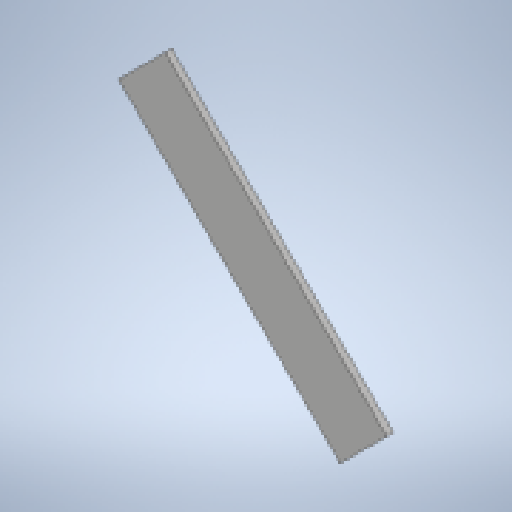
# Autodesk Inventor part: CameraPlate
Saved by Autodesk Inventor 2025.1 (Build 291241000, 241)
## iProperties
Created: 2025-06-16
Part Number: CameraPlate
Material: Generic
Document SubType Name: Modeling
Designer: User
Density: 1 g/cm^3
Appearance: Default
Author: User
Autodesk Inventor part; units mm, degrees
ref_plane "YZ Plane" through (0, 0, 0) normal (1, 0, 0) x (0, 1, 0)
ref_plane "XZ Plane" through (0, 0, 0) normal (0, 1, 0) x (-1, 0, 0)
ref_plane "XY Plane" through (0, 0, 0) normal (0, 0, 1) x (1, 0, 0)
sketch "Sketch3" plane through (0, 0, 0) normal (0, 0, 1) x (1, 0, 0)
  line L0 (-94.6243, 4.4908) -> (-47.5665, 51.5485) projected
  line L1 (-48.2912, 50.8239) -> (-38.3917, 60.7234) projected
  line L2 (-39.1164, 59.9987) -> (15.6159, 114.7309) projected
  line L3 (75.9757, -27.3497) -> (-17.6132, -120.9386) projected
  line L4 (-13.085, -29.4897) -> (-26.753, -15.8218) projected
  line L5 (-9.5495, -25.9542) -> (-23.2174, -12.2862)
  line L6 (33.9109, -69.4145) -> (-67.3094, 31.8057)
  line L7 (-67.3094, 31.8057) -> (-46.0962, 53.0189)
  line L8 (-46.0962, 53.0189) -> (55.1241, -48.2013)
  line L9 (55.1241, -48.2013) -> (33.9109, -69.4145)
  point P0 (0, 0)
  point P1 (55.1241, -48.2013)
  dimension "d0" = 5
  dimension "d1" = 30
  constraints: 10 end point, 3 parallel, 2 perpendicular, 2 point on line
  measures "d0" distance between parallel lines of L4 L5
  measures "d1" distance of L6.end L7.end
extrude "Extrusion1" add sketch "Sketch3" along normal blind 3
sketch "Sketch4" plane through (0, 0, 3) normal (0, 0, 1) x (1, 0, 0)
  line L0 (-37.1973, -4.3252) -> (-44.2684, 2.7459) projected
  line L1 (4.8755, -46.3981) -> (-2.1956, -39.327) projected
  line L2 (-67.3094, 31.8057) -> (33.9109, -69.4145) projected
  line L3 (-13.085, -29.4897) -> (-26.753, -15.8218) projected
  line L4 (-44.125, 2.6025) -> (-37.1973, -4.3252)
  line L5 (-37.1973, -4.3252) -> (-34.1879, -1.3158)
  line L6 (-34.1879, -1.3158) -> (-41.1156, 5.6119)
  line L7 (-41.1156, 5.6119) -> (-44.125, 2.6025)
  line L8 (-2.1956, -39.327) -> (4.8755, -46.3981)
  line L9 (4.8755, -46.3981) -> (7.8849, -43.3886)
  line L10 (7.8849, -43.3886) -> (0.8139, -36.3176)
  line L11 (0.8139, -36.3176) -> (-2.1956, -39.327)
  point P0 (0, 0)
  constraints: 16 end point, 4 parallel, 2 collinear, 2 perpendicular, 1 point on line
extrude "Extrusion2" add sketch "Sketch4" against normal up to surface (3 mm away)
sketch "Sketch5" plane through (0, 0, 3) normal (0, 0, 1) x (1, 0, 0)
  line L0 (-19.5198, 27.4945) -> (-12.4488, 20.4234) projected
  line L1 (22.553, -14.5784) -> (29.6241, -21.6495) projected
  line L2 (55.1241, -48.2013) -> (-46.0962, 53.0189) projected
  line L3 (-12.4488, 20.4234) -> (-19.5198, 27.4945)
  line L4 (-19.5198, 27.4945) -> (-20.0458, 26.9685)
  line L5 (-20.0458, 26.9685) -> (-12.9747, 19.8974)
  line L6 (-12.9747, 19.8974) -> (-12.4488, 20.4234)
  line L7 (29.6241, -21.6495) -> (22.553, -14.5784)
  line L8 (22.553, -14.5784) -> (22.0271, -15.1043)
  line L9 (22.0271, -15.1043) -> (29.0981, -22.1754)
  line L10 (29.0981, -22.1754) -> (29.6241, -21.6495)
  point P0 (0, 0)
  constraints: 16 end point, 5 parallel, 2 perpendicular, 1 collinear
extrude "Extrusion3" add sketch "Sketch5" against normal up to surface (3 mm away)
sketch "Sketch6" plane through (0, 0, 3) normal (0, 0, 1) x (1, 0, 0)
  ellipse E0 centre (-19.5198, 20.4234) end of major axis (-20.5805, 21.4841) minor radius 1.5 projected
  ellipse E1 centre (-37.1974, 2.7458) end of major axis (-38.258, 3.8065) minor radius 1.5 projected
  ellipse E2 centre (22.5531, -21.6494) end of major axis (21.4924, -20.5888) minor radius 1.5 projected
  ellipse E3 centre (4.8755, -39.327) end of major axis (3.8148, -38.2663) minor radius 1.5 projected
  point P0 (0, 0)
  constraints: 4 other
extrude "Extrusion4" cut sketch "Sketch6" against normal blind 10
sketch "Sketch8" plane through (0, 0, 0) normal (0, 0, -1) x (-1, 0, 0)
  line L0 (53.1672, 45.9478) -> (-48.053, -55.2724)
  line L1 (60.2383, 38.8768) -> (-40.9819, -62.3435)
  line L2 (61.0868, 38.0282) -> (-40.1334, -63.192)
  line L3 (59.3898, 39.7253) -> (-41.8305, -61.4949)
  line L4 (52.3187, 46.7964) -> (-48.9015, -54.4239)
  line L5 (54.0158, 45.0993) -> (-47.2045, -56.1209)
  line L6 (61.0868, 38.0282) -> (59.3898, 39.7253)
  line L7 (54.0158, 45.0993) -> (52.3187, 46.7964)
  line L8 (-40.1334, -63.192) -> (-41.8305, -61.4949)
  line L9 (-47.2045, -56.1209) -> (-48.9015, -54.4239)
  line L10 (-33.9109, -69.4145) -> (-55.1241, -48.2013) projected
  point P0 (0, 0)
  point P1 (46.0962, 53.0189)
  point P2 (67.3094, 31.8057)
  dimension "d16" = 1.2
  dimension "d17" = 1.2
  dimension "d18" = 1.2
  dimension "d19" = 1.2
  constraints: 20 end point, 4 parallel, 2 collinear, 2 perpendicular
  measures "d16" distance between parallel lines of L1 L2
  measures "d17" distance between parallel lines of L1 L3
  measures "d18" distance between parallel lines of L0 L4
  measures "d19" distance between parallel lines of L0 L5
extrude "Extrusion6" add sketch "Sketch8" along normal blind 5
chamfer "Chamfer1" distance 0.73 angle 45 4 edges at (29.0981, -22.1754, 1.5) (22.0271, -15.1043, 1.5) (-20.0458, 26.9685, 1.5) (-12.9747, 19.8974, 1.5)
chamfer "Chamfer2" distance 4.25 angle 45 4 edges at (-41.1156, 5.6119, 1.5) (-34.1879, -1.3158, 1.5) (7.8849, -43.3886, 1.5) (0.8139, -36.3176, 1.5)
sketch "Sketch9" plane through (-67.3094, 31.8057, 0) normal (-0.7071068, 0.7071068, 0) x (-0.7071068, -0.7071068, 0)
  line L0 (-30, 0) -> (-21.2, 0) projected
  line L1 (-21.2, 0) -> (-21.2, -5) projected
  line L2 (-18.8, -5) -> (-21.2, -5) projected
  line L3 (-18.8, 0) -> (-18.8, -5) projected
  line L4 (-18.8, 0) -> (-11.2, 0) projected
  line L5 (-11.2, 0) -> (-11.2, -5) projected
  line L6 (-8.8, -5) -> (-11.2, -5) projected
  line L7 (-8.8, 0) -> (-8.8, -5) projected
  line L8 (-8.8, 0) -> (0, 0) projected
  line L9 (0, 0) -> (0, 3) projected
  line L10 (-30, 3) -> (0, 3) projected
  line L11 (-30, 0) -> (-30, 3) projected
  line L12 (-30, 3) -> (0, 3)
  line L13 (0, 3) -> (0, 0)
  line L14 (0, 0) -> (-30, 0)
  line L15 (-30, 0) -> (-30, 3)
  point P0 (-25.1049, 0)
  constraints: 8 end point, 2 parallel, 1 horizontal, 1 perpendicular
extrude "Extrusion7" add sketch "Sketch9" along normal blind 13 contours L11 L10 L9 L8 L14 L4 L0
sketch "Sketch10" plane through (55.1241, -48.2013, 3) normal (0.7071068, -0.7071068, 0) x (-0.7071068, -0.7071068, 0)
  line L0 (30, 3) -> (30, 0) projected
  line L1 (0, 3) -> (-0.73, 3) projected
  line L2 (30, 0) -> (-0.73, 0)
  line L3 (-0.73, 0) -> (-0.73, 3)
  line L4 (-0.73, 3) -> (30, 3)
  line L5 (30, 3) -> (30, 0)
  line L6 (30, 3) -> (21.2, 3) projected
  line L7 (21.2, 3) -> (21.2, 8) projected
  line L8 (18.8, 8) -> (21.2, 8) projected
  line L9 (18.8, 3) -> (18.8, 8) projected
  line L10 (18.8, 3) -> (11.2, 3) projected
  line L11 (11.2, 3) -> (11.2, 8) projected
  line L12 (8.8, 8) -> (11.2, 8) projected
  line L13 (8.8, 3) -> (8.8, 8) projected
  line L14 (8.8, 3) -> (0, 3) projected
  line L15 (0, 3) -> (0, 0) projected
  line L16 (30, 0) -> (0, 0) projected
  line L17 (30, 3) -> (30, 0) projected
  line L18 (8.8, 3) -> (0, 3) projected
  line L19 (30, 0) -> (0, 0) projected
  line L20 (0, 3) -> (30, 3)
  line L21 (30, 3) -> (30, 0)
  line L22 (30, 0) -> (0, 0)
  line L23 (0, 0) -> (0, 3)
  point P0 (4.8951, 3)
  point P1 (0, 3)
  point P2 (0, 3)
  constraints: 16 end point, 4 parallel, 2 horizontal, 2 perpendicular
extrude "Extrusion8" add sketch "Sketch10" along normal blind 13 contours L0 L2 L15 L4
sketch "Sketch11" plane through (0, 0, 3) normal (0, 0, 1) x (1, 0, 0)
  line L0 (-54.0158, 45.0993) -> (-52.3187, 46.7964) projected
  line L1 (-61.0868, 38.0282) -> (-59.3898, 39.7253) projected
  ellipse E0 centre (4.8755, -39.327) end of major axis (3.8148, -38.2663) minor radius 1.5 projected
  ellipse E1 centre (-37.1974, 2.7458) end of major axis (-38.258, 3.8065) minor radius 1.5 projected
  ellipse E2 centre (22.5531, -21.6494) end of major axis (21.4924, -20.5888) minor radius 1.5 projected
  ellipse E3 centre (-19.5198, 20.4234) end of major axis (-20.5805, 21.4841) minor radius 1.5 projected
  line L2 (-44.1208, 8.6171) -> (-76.5018, 40.9981) projected
  line L3 (-44.1208, 2.6067) -> (-44.1208, 8.6171) projected
  line L4 (-44.1208, 2.6067) -> (-44.125, 2.6025) projected
  line L5 (-44.125, 2.6025) -> (-37.1973, -4.3252) projected
  line L6 (-37.1973, -4.3252) -> (-37.1931, -4.321) projected
  line L7 (-31.1827, -4.321) -> (-37.1931, -4.321) projected
  line L8 (-31.1827, -4.321) -> (-2.1913, -33.3123) projected
  line L9 (-2.1913, -39.3228) -> (-2.1913, -33.3123) projected
  line L10 (-2.1913, -39.3228) -> (-2.1956, -39.327) projected
  line L11 (-2.1956, -39.327) -> (4.8755, -46.3981) projected
  line L12 (4.8755, -46.3981) -> (4.8797, -46.3938) projected
  line L13 (10.8901, -46.3938) -> (4.8797, -46.3938) projected
  line L14 (10.8901, -46.3938) -> (43.1032, -78.6069) projected
  line L15 (64.3165, -57.3937) -> (43.1032, -78.6069) projected
  line L16 (29.6143, -22.6916) -> (64.3165, -57.3937) projected
  line L17 (29.6143, -21.6592) -> (29.6143, -22.6916) projected
  line L18 (29.6143, -21.6592) -> (29.6241, -21.6495) projected
  line L19 (29.6241, -21.6495) -> (22.553, -14.5784) projected
  line L20 (22.553, -14.5784) -> (22.5433, -14.5882) projected
  line L21 (21.5109, -14.5882) -> (22.5433, -14.5882) projected
  line L22 (21.5109, -14.5882) -> (-12.4585, 19.3813) projected
  line L23 (-12.4585, 20.4136) -> (-12.4585, 19.3813) projected
  line L24 (-12.4585, 20.4136) -> (-12.4488, 20.4234) projected
  line L25 (-12.4488, 20.4234) -> (-19.5198, 27.4945) projected
  line L26 (-19.5198, 27.4945) -> (-19.5296, 27.4847) projected
  line L27 (-20.562, 27.4847) -> (-19.5296, 27.4847) projected
  line L28 (-20.562, 27.4847) -> (-55.2886, 62.2113) projected
  line L29 (-76.5018, 40.9981) -> (-55.2886, 62.2113) projected
  line L30 (75.9757, -27.3497) -> (-17.6132, -120.9386) projected
  circle A0 centre (43.1032, -69.4145) radius 6.5
  circle A1 centre (55.1241, -57.3937) radius 6.5
  line L31 (-76.5018, 40.9981) -> (-67.3094, 31.8057)
  line L32 (-67.3094, 31.8057) -> (-46.0962, 53.0189)
  line L33 (-46.0962, 53.0189) -> (-55.2886, 62.2113)
  line L34 (-55.2886, 62.2113) -> (-76.5018, 40.9981)
  circle A2 centre (-67.3094, 40.9981) radius 6.5
  circle A3 centre (-55.2886, 53.0189) radius 6.5
  circle A4 centre (-67.3094, 40.9981) radius 1.5
  circle A5 centre (-55.2886, 53.0189) radius 1.5
  circle A6 centre (43.1032, -69.4145) radius 1.5
  circle A7 centre (55.1241, -57.3937) radius 1.5
  point P0 (0, 0)
  point P1 (47.6994, -74.0107)
  point P2 (38.5071, -74.0107)
  point P3 (59.7203, -52.7975)
  point P4 (59.7203, -61.9899)
  point P5 (-59.8848, 57.6151)
  point P6 (-50.6924, 57.6151)
  point P7 (-71.9056, 36.4019)
  point P8 (-71.9056, 45.5943)
  dimension "d32" = 3
  dimension "d33" = 3
  dimension "d34" = 3
  dimension "d35" = 3
  constraints: 12 tangent, 8 centre point, 8 end point, 4 coincident, 2 parallel, 1 perpendicular, 1 point on line, 4 other
  measures "d32" diameter of A4
  measures "d33" diameter of A5
  measures "d34" diameter of A6
  measures "d35" diameter of A7
extrude "Extrusion9" cut sketch "Sketch11" against normal blind 13 contours L29 L28 A3 | A2 L2 L29 | L16 L15 A1 | A0 L15 L14 | A4 | A5 | A6 | A7
body "Solid1"
